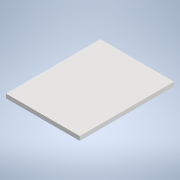
# Autodesk Inventor part: platformm
Saved by Autodesk Inventor 2022 (Build 260153070, 153G)
## iProperties
Created: 2021-07-24
Part Number: platformm
Material: Generic
Document SubType Name: Modeling
Designer: sachin
Density: 1 g/cm^3
Appearance: Default
Author: sachin
Autodesk Inventor part; units mm, degrees
ref_plane "YZ Plane" through (0, 0, 0) normal (1, 0, 0) x (0, 1, 0)
ref_plane "XZ Plane" through (0, 0, 0) normal (0, 1, 0) x (-1, 0, 0)
ref_plane "XY Plane" through (0, 0, 0) normal (0, 0, 1) x (1, 0, 0)
sketch "Sketch1" plane through (0, 0, 0) normal (0, 1, 0) x (-1, 0, 0)
  line L0 (246.1921, 473.481) -> (-338.0079, 473.481)
  line L1 (-338.0079, 473.481) -> (-338.0079, -110.719)
  line L2 (-338.0079, -110.719) -> (246.1921, -110.719)
  line L3 (246.1921, -110.719) -> (246.1921, 473.481)
  point P0 (0, 0)
  dimension "d0" = 584.2
  dimension "d1" = 584.2
  constraints: 8 end point, 2 parallel, 1 horizontal, 1 perpendicular
  measures "d0" distance of L2.end L0.start
  measures "d1" distance of L1.end L2.end
extrude "Extrusion1" add sketch "Sketch1" along normal blind 25.4
sketch "Sketch2" plane through (-246.1921, 0, -110.719) normal (-1, 0, 0) x (0, 0, 1)
  line L0 (584.2, 25.4) -> (0, 25.4) projected
  line L1 (584.2, 0) -> (0, 0) projected
  line L2 (0, 25.4) -> (584.2, 25.4)
  line L3 (584.2, 25.4) -> (584.2, 0)
  line L4 (584.2, 0) -> (0, 0)
  line L5 (0, 0) -> (0, 25.4)
  point P0 (110.719, 0)
  point P1 (0, 0)
  constraints: 8 end point, 2 parallel, 1 horizontal, 1 perpendicular
extrude "Extrusion2" add sketch "Sketch2" along normal blind 76.2
body "Solid1"
